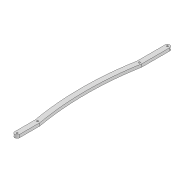
# Autodesk Inventor part: Part_5
Saved by Autodesk Inventor 2022 (Build 260153000, 153)
## iProperties
Created: 2022-04-22
Part Number: Part_5
Material: Generic
Document SubType Name: Modeling
Designer: dell
Density: 1 g/cm^3
Appearance: Default
Mass: 3.80646 g
Surface Area: 32.1371 cm^2
Volume: 3.80646 cm^3
Author: dell
Autodesk Inventor part; units mm, degrees
ref_plane "YZ Plane" through (0, 0, 0) normal (1, 0, 0) x (0, 1, 0)
ref_plane "XZ Plane" through (0, 0, 0) normal (0, 1, 0) x (-1, 0, 0)
ref_plane "XY Plane" through (0, 0, 0) normal (0, 0, 1) x (1, 0, 0)
sketch "Sketch1" plane through (0, 0, 0) normal (0, 1, 0) x (-1, 0, 0)
  line L0 (0, 0) -> (0, -312.648) construction
  line L1 (5, 0) -> (5, -312.648)
  line L2 (-5, -312.648) -> (-5, 0)
  arc A0 (5, 0) -> (-5, 0) centre (0, 0) ccw
  arc A1 (-5, -312.648) -> (5, -312.648) centre (0, -312.648) ccw
  circle A2 centre (0, 0) radius 1.65
  circle A3 centre (0, -312.648) radius 1.65
  circle A4 centre (0, -42.6) radius 1.65
  circle A5 centre (0, -254.274) radius 1.65
  arc A6 (5, -254.274) -> (5, -42.6) centre (-585.5917, -148.437) ccw
  arc A7 (-5, -254.274) -> (-5, -42.6) centre (-595.5917, -148.437) ccw
  point P0 (0, -156.324)
  dimension "d0" = 3.3
  dimension "d1" = 3.3
  dimension "d2" = 10
  dimension "d3" = 312.648
  dimension "d10" = 3.3
  dimension "d11" = 42.6
  dimension "d12" = 3.3
  dimension "d13" = 254.274
  dimension "d16" = 600
  dimension "d17" = 600
  constraints: 8 centre point, 8 end point, 8 point on circle, 6 point on line, 4 horizontal alignment, 4 tangent, 2 coincident, 1 midpoint, 1 parallel, 1 vertical
  measures "d0" diameter of A2
  measures "d1" diameter of A3
  measures "d2" distance between parallel lines of L2 L1
  measures "d3" distance of L0.end L0.start
  measures "d10" diameter of A4
  measures "d11" distance of L0.start A4.centre
  measures "d12" diameter of A5
  measures "d13" distance of L0.start A5.centre
  measures "d16" radius of A6
  measures "d17" radius of A7
extrude "Extrusion1" add sketch "Sketch1" along normal blind 6 contours L1 A1 L2 A7 A0 | A6 L1
body "Solid1"
